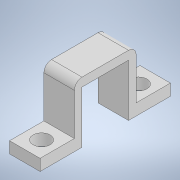
# Autodesk Inventor part: Linear Actuator Mount
Saved by Autodesk Inventor 2021 (Build 250183000, 183)
## iProperties
Created: 2021-06-25
Part Number: Linear Actuator Mount
Material: Generic
Document SubType Name: Modeling
Designer: Work
Density: 1 g/cm^3
Appearance: Default
Author: Work
Autodesk Inventor part; units mm, degrees
ref_plane "YZ Plane" through (0, 0, 0) normal (1, 0, 0) x (0, 1, 0)
ref_plane "XZ Plane" through (0, 0, 0) normal (0, 1, 0) x (-1, 0, 0)
ref_plane "XY Plane" through (0, 0, 0) normal (0, 0, 1) x (1, 0, 0)
sketch "Sketch1" plane through (0, 0, 0) normal (1, 0, 0) x (0, 1, 0)
  line L0 (0, 0) -> (3, 0)
  line L1 (3, 0) -> (3, -8.5)
  line L2 (3, -25.7) -> (3, -34.2)
  line L3 (3, -34.2) -> (0, -34.2)
  line L4 (0, -34.2) -> (0, -25.7)
  line L5 (0, -25.7) -> (0, -23.2)
  line L6 (0, -23.2) -> (13.7, -23.2)
  line L7 (0, 0) -> (0, -8.5)
  line L8 (0, -8.5) -> (0, -11)
  line L9 (0, -11) -> (13.7, -11)
  line L10 (13.7, -11) -> (13.7, -23.2)
  line L11 (3, -8.5) -> (3, -9)
  line L12 (3, -25.7) -> (3, -25.2)
  line L13 (3, -9) -> (15.95, -9)
  line L14 (3, -25.2) -> (15.95, -25.2)
  line L15 (15.95, -25.2) -> (15.95, -9)
  dimension "d0" = 3
  dimension "d1" = 8.5
  dimension "d4" = 8.5
  dimension "d8" = 3
  dimension "d12" = 13.7
  dimension "d14" = 12.2
  dimension "d28" = 0.5
  dimension "d29" = 0.5
  dimension "d30" = 2.25
  constraints: 32 end point, 6 perpendicular, 4 vertical, 3 horizontal, 2 point on line
  measures "d0" distance of L0.start L0.end
  measures "d1" distance of L0.end L1.end
  measures "d4" distance of L2.start L2.end
  measures "d8" distance between parallel lines of L4 L2
  measures "d12" distance from line of L5.end L10
  measures "d14" distance between parallel lines of L6 L9
  measures "d28" distance of L1.end L11.end
  measures "d29" distance of L2.start L12.end
  measures "d30" distance between parallel lines of L10 L15
extrude "Extrusion1" add sketch "Sketch1" against normal blind 8
sketch "Sketch3" plane through (0, 3, 0) normal (0, 1, 0) x (1, 0, 0)
  circle A0 centre (-4, 29.8) radius 2.25
  line L0 (0, 34.2) -> (-8, 34.2) projected
  line L1 (0, 34.2) -> (0, 25.2) projected
  line L2 (0, 0) -> (-8, 0) projected
  line L3 (0, 9) -> (0, 0) projected
  circle A1 centre (-4, 4.4) radius 2.25
  point P0 (0, 25.8)
  point P1 (0, 8.5)
  dimension "d16" = 4.5
  dimension "d18" = 4.4
  dimension "d19" = 4
  dimension "d23" = 4.5
  dimension "d24" = 4
  dimension "d25" = 4.4
  constraints: 2 centre point
  measures "d16" diameter of A0
  measures "d18" distance from line of L0 A0.centre
  measures "d19" distance from line of L1 A0.centre
  measures "d23" diameter of A1
  measures "d24" distance from line of L3 A1.centre
  measures "d25" distance from line of L2 A1.centre
extrude "Extrusion2" cut sketch "Sketch3" against normal through all
fillet "Fillet1" radius 2 2 edges at (-4, 15.95, -9) (-4, 15.95, -25.2)
body "Solid1"
